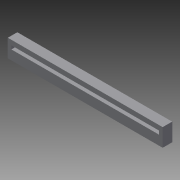
# Autodesk Inventor part: bottom_board_slat_back
Saved by Autodesk Inventor 2014 SP1 (Build 180222100, 222)
## iProperties
Created: 2014-02-20
Part Number: bottom_board_slat_back
Material: Wood (Birch)
Document SubType Name: Modeling
Designer: Chris
Density: 0.55 g/cm^3
Appearance: Birch - Natural Polished
Mass: 254.966 g
Surface Area: 703.829 cm^2
Volume: 463.575 cm^3
Author: Chris
Autodesk Inventor part; units mm, degrees
ref_plane "YZ Plane" through (0, 0, 0) normal (1, 0, 0) x (0, 1, 0)
ref_plane "XZ Plane" through (0, 0, 0) normal (0, 1, 0) x (-1, 0, 0)
ref_plane "XY Plane" through (0, 0, 0) normal (0, 0, 1) x (1, 0, 0)
sketch "Sketch1" plane through (0, 0, 0) normal (0, 0, 1) x (1, 0, 0)
  line L0 (0, 0) -> (-412.75, 0)
  line L1 (-412.75, 0) -> (-412.75, 47.625)
  line L2 (-412.75, 47.625) -> (0, 47.625)
  line L3 (0, 47.625) -> (0, 0)
  dimension "d0" = 412.75
  dimension "d1" = 47.625
  constraints: 8 end point, 2 parallel, 1 horizontal, 1 perpendicular
  measures "d0" distance of L1.end L2.end
  measures "d1" distance of L2.end L0.start
extrude "Extrusion1" add sketch "Sketch1" against normal blind 25.4
sketch "Sketch2" plane through (0, 0, 0) normal (0, 0, 1) x (1, 0, 0)
  line L0 (0, 47.625) -> (0, 0) projected
  line L1 (-412.75, 47.625) -> (0, 47.625) projected
  line L2 (-412.75, 0) -> (-412.75, 47.625) projected
  line L3 (-403.225, 34.925) -> (-9.525, 34.925)
  line L4 (-9.525, 34.925) -> (-9.525, 25.4)
  line L5 (-9.525, 25.4) -> (-403.225, 25.4)
  line L6 (-403.225, 25.4) -> (-403.225, 34.925)
  line L7 (0, 0) -> (-412.75, 0) projected
  dimension "d4" = 12.7
  dimension "d5" = 9.525
  dimension "d10" = 412.75
  dimension "d12" = 25.4
  dimension "d14" = 9.525
  dimension "d16" = 9.525
  constraints: 8 end point, 2 parallel, 1 horizontal, 1 perpendicular
  measures "d4" distance between parallel lines of L1 L3
  measures "d5" distance of L5.end L3.start
  measures "d10" distance of L1.start L0.start
  measures "d12" distance from line of L7 L4.end
  measures "d14" distance between parallel lines of L6 L2
  measures "d16" distance between parallel lines of L0 L4
extrude "Extrusion2" cut sketch "Sketch2" against normal blind 9.525 contours L3 L4 L5 L6
equation "\"d16\" = d14"
body "Solid1"
